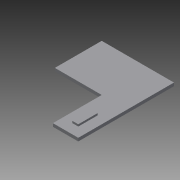
# Autodesk Inventor part: sensores
Saved by Autodesk Inventor 2015 SP1 (Build 190203100, 203)
## iProperties
Created: 2015-06-09
Part Number: sensores
Material: Generic
Document SubType Name: Modeling
Designer: pc
Density: 1 g/cm^3
Appearance: Default
Author: pc
Autodesk Inventor part; units mm, degrees
ref_plane "YZ Plane" through (0, 0, 0) normal (1, 0, 0) x (0, 1, 0)
ref_plane "XZ Plane" through (0, 0, 0) normal (0, 1, 0) x (-1, 0, 0)
ref_plane "XY Plane" through (0, 0, 0) normal (0, 0, 1) x (1, 0, 0)
sketch "Sketch1" plane through (0, 0, 0) normal (0, 0, 1) x (1, 0, 0)
  line L0 (-18.5577, 19.3606) -> (18.4423, 19.3606)
  line L1 (18.4423, 19.3606) -> (18.4423, -29.6394)
  line L2 (18.4423, -29.6394) -> (5.4423, -29.6394)
  line L3 (5.4423, -29.6394) -> (5.4423, -4.6394)
  line L4 (5.4423, -4.6394) -> (-18.5577, -4.6394)
  line L5 (-18.5577, -4.6394) -> (-18.5577, 19.3606)
  point P0 (0, 0)
  dimension "d0" = 37
  dimension "d1" = 49
  dimension "d2" = 13
  dimension "d3" = 24
  constraints: 13 end point, 3 perpendicular, 1 horizontal
  measures "d0" distance of L0.start L0.end
  measures "d1" distance of L0.end L1.end
  measures "d2" distance of L1.end L2.end
  measures "d3" distance of L4.end L0.start
extrude "Extrusion1" add sketch "Sketch1" along normal blind 1.6
sketch "Sketch2" plane through (0, 0, 1.6) normal (0, 0, 1) x (1, 0, 0)
  line L0 (18.4423, 19.3606) -> (-18.5577, 19.3606) projected
  line L1 (-18.5577, 19.3606) -> (-18.5577, -4.6394) projected
  line L2 (-18.5577, -4.6394) -> (5.4423, -4.6394) projected
  line L3 (5.4423, -4.6394) -> (5.4423, -29.6394) projected
  line L4 (5.4423, -29.6394) -> (18.4423, -29.6394) projected
  line L5 (18.4423, -29.6394) -> (18.4423, 19.3606) projected
  line L6 (10.4423, -14.6394) -> (13.4423, -14.6394)
  line L7 (13.4423, -14.6394) -> (13.4423, -24.6394)
  line L8 (13.4423, -24.6394) -> (10.4423, -24.6394)
  line L9 (10.4423, -24.6394) -> (10.4423, -14.6394)
  point P0 (0, 0)
  dimension "d9" = 3
  dimension "d10" = 10
  dimension "d11" = 5
  dimension "d14" = 5
  constraints: 8 end point, 2 parallel, 1 horizontal, 1 perpendicular
  measures "d9" distance of L7.end L8.end
  measures "d10" distance of L6.end L7.end
  measures "d11" horizontal distance of L3.end L8.end
  measures "d14" horizontal distance of L3.end L8.end
extrude "Extrusion2" add sketch "Sketch2" along normal blind 1 contours L6 L7 L8 L9
body "Solid1"
